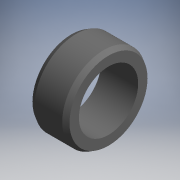
# Autodesk Inventor part: 150927 ZBH-9
Saved by Autodesk Inventor 2017.3 (Build 213256000, 256)
## iProperties
Part Number: 150927 ZBH-9
Material: Generic
Catalog Web Link: www.cadenas.de
Description: ZBH-centring sleeve
Vendor: FESTO
Document SubType Name: Modeling
Designer: partserver
Manufacturer: FESTO
Mass: 0.121796 g
Surface Area: 2.43943 cm^2
Volume: 0.121796 cm^3
Density: 1 g/cm^3
Appearance: PSOLRGB-128-128-128
Category: PARTsolutions
Company: FESTO
Title: 150927 ZBH-9
Author: Cadenas PARTsolutions
Comments: centring sleeve
PSOL_IDENT_0: {$CADENAS_DATA\23d-libs\festo\parts\z\zbh\zbh.prj},161 {VTYP=3D},{NB=150927 ZBH-9},{LINA=150927 ZBH-
PSOL_IDENT_1: 9},{NN=ZBH},{DATE=24.04.2020 12:36:33},{GEOMDATE=24.04.2020 12:01:39},{VERSION=},{LINEID=30},{WBVAR=
PSOL_IDENT_2: },{WBNUMERIC=}  {NB=150927 ZBH-9},{LINA=150927 ZBH-9},{KT=DUMMY},{TNR=150927},{TYP=ZBH-9},{B1=4.000}
PSOL_IDENT_3: ,{D1=9.000},{D2=6.400},{CNSMASSEXACT=0.000}
NB: 150927 ZBH-9
NN: ZBH
NT: centring sleeve
NBSYN: $TNR. $TYP.
LINA: 150927 ZBH-9
CATALOG: Festo
TNR: 150927
TYP: ZBH-9
B1: 4
D1: 9
D2: 6.4
CNSMASSEXACT: 0
SUPPLIER: FESTO
ARTICLENO: 150927 ZBH-9
BOMINFO: 150927 ZBH-9
CREATOR: CADENAS GmbH
Autodesk Inventor part; units mm, degrees
sketch "Sketch_1" plane through (0, 0, 0) normal (0, 0, 1) x (1, 0, 0)
  line L0 (4, 0) -> (0, 0)
  line L1 (0, 3.2) -> (4, 3.2)
  line L2 (4, 3.2) -> (4, 4.2113)
  line L3 (4, 4.2113) -> (3.5, 4.5)
  line L4 (3.5, 4.5) -> (0.5, 4.5)
  line L5 (0.5, 4.5) -> (0, 4.2113)
  line L6 (0, 4.2113) -> (0, 3.2)
  constraints: 14 end point
revolve "Revolution1" add sketch "Sketch_1" angle 360 about axis through (4, 0, 0) along (-1, 0, 0)
ref_plane "anbau_XY" through (0, 0, 0) normal (1, 0, 0) x (0, 0, -1)
ref_plane "anbau_YZ" through (0, 0, 0) normal (0, 0, -1) x (0, 1, 0)
ref_plane "anbau_ZX" through (0, 0, 0) normal (0, 1, 0) x (1, 0, 0)
ref_plane "insert_XY" through (0, 0, 0) normal (1, 0, 0) x (0, 0, -1)
ref_plane "insert_YZ" through (0, 0, 0) normal (0, 0, -1) x (0, 1, 0)
ref_plane "insert_ZX" through (0, 0, 0) normal (0, 1, 0) x (1, 0, 0)
ref_plane "schraube_punkt_XY" through (4, 0, 0) normal (1, 0, 0) x (0, 0, -1)
ref_plane "schraube_punkt_YZ" through (4, 0, 0) normal (0, 0, -1) x (0, 1, 0)
ref_plane "schraube_punkt_ZX" through (4, 0, 0) normal (0, 1, 0) x (1, 0, 0)
body "Solid1"
